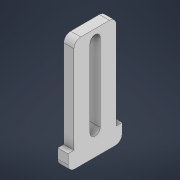
# Autodesk Inventor part: Ga motor 1
Saved by Autodesk Inventor 2021 (Build 250183000, 183)
## iProperties
Created: 2022-03-15
Part Number: Ga motor 1
Material: Generic
Document SubType Name: Modeling
Designer: phand
Density: 1 g/cm^3
Appearance: Default
Author: phand
Autodesk Inventor part; units mm, degrees
ref_plane "YZ Plane" through (0, 0, 0) normal (1, 0, 0) x (0, 1, 0)
ref_plane "XZ Plane" through (0, 0, 0) normal (0, 1, 0) x (-1, 0, 0)
ref_plane "XY Plane" through (0, 0, 0) normal (0, 0, 1) x (1, 0, 0)
sketch "Sketch1" plane through (0, 0, 0) normal (1, 0, 0) x (0, 1, 0)
  line L0 (-11.6, 8) -> (-14.5, 8)
  line L1 (-16.5, 6) -> (-16.5, -6)
  line L2 (-14.5, -8) -> (-11.6, -8)
  line L3 (16.5, 8) -> (-16.5, -8) construction
  line L4 (-11.6, 8) -> (-11.6, 6.25)
  line L5 (-11.6, 6.25) -> (14.4, 6.25)
  line L6 (-11.6, -6.25) -> (14.4, -6.25)
  line L7 (-11.6, 8) -> (-11.6, 6.25)
  line L8 (-11.6, -6.25) -> (-11.6, -8)
  arc A0 (-14.5, 8) -> (-16.5, 6) centre (-14.5, 6) ccw
  arc A1 (-16.5, -6) -> (-14.5, -8) centre (-14.5, -6) ccw
  line L9 (-16.5, 8) -> (-3.0507, 1.4791) construction
  line L10 (-2.2931, 1.1118) -> (16.5, -8) construction
  arc A2 (13.4, -1.5) -> (13.4, 1.5) centre (13.4, 0) ccw
  arc A3 (-9.6, 1.5) -> (-9.6, -1.5) centre (-9.6, 0) ccw
  line L11 (13.4, 1.5) -> (-9.6, 1.5)
  line L12 (-9.6, -1.5) -> (13.4, -1.5)
  line L13 (16.4, 4.25) -> (16.4, -4.25)
  arc A4 (16.4, 4.25) -> (14.4, 6.25) centre (14.4, 4.25) ccw
  arc A5 (14.4, -6.25) -> (16.4, -4.25) centre (14.4, -4.25) ccw
  point P0 (16.4, 6.25)
  point P1 (16.4, -6.25)
  dimension "d1" = 16
  dimension "d3" = 1.75
  dimension "d5" = 2
  dimension "d14" = 1.75
  dimension "d18" = 3
  dimension "d19" = 3
  dimension "d21" = 2
  dimension "d24" = 28
  dimension "d25" = 2
  constraints: 28 end point, 12 point on circle, 10 tangent, 8 point on line, 6 centre point, 3 perpendicular, 2 equal radius, 2 horizontal, 1 parallel, 1 vertical
  measures "d1" distance of L10.end L3.start
  measures "d3" distance of L4.end L0.start
  measures "d5" radius of A0
  measures "d14" distance of L6.start L2.end
  measures "d18" diameter of A2
  measures "d19" diameter of A3
  measures "d21" distance from line of L8 A3.centre
  measures "d24" distance of L4.end point (16.4, 6.25)
  measures "d25" radius of A4
extrude "Extrusion3" add sketch "Sketch1" along normal blind 3
body "Solid3"
